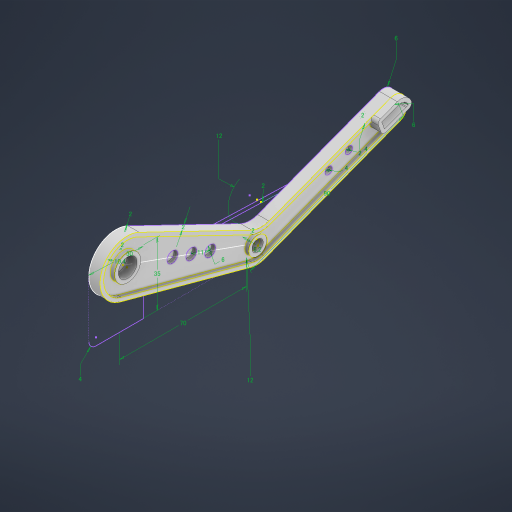
# Autodesk Inventor part: myPartbasic
Saved by Autodesk Inventor 2024.3 (Build 283343000, 343)
## iProperties
Created: 2024-11-22
Part Number: myPartbasic
Material: 一般
Document SubType Name: Modeling
Designer: ktamu
Density: 1 g/cm^3
Appearance: 既定
Author: ktamu
Autodesk Inventor part; units mm, degrees
ref_plane "YZ Plane" through (0, 0, 0) normal (1, 0, 0) x (0, 1, 0)
ref_plane "XZ Plane" through (0, 0, 0) normal (0, 1, 0) x (-1, 0, 0)
ref_plane "XY Plane" through (0, 0, 0) normal (0, 0, 1) x (1, 0, 0)
sketch "スケッチ1" plane through (0, 0, 0) normal (1, 0, 0) x (0, 1, 0)
  circle A0 centre (0, 0) radius 5.2
  circle A1 centre (0, 0) radius 7.2
  circle A2 centre (0, 0) radius 15
  line L0 (0, 15) -> (0, -15)
  line L1 (0, -15) -> (-35, -15)
  line L2 (-35, -15) -> (-35, 11)
  line L3 (-31, 15) -> (0, 15) construction
  line L4 (-35, -2) -> (-35, -69.78961) construction
  line L5 (-16.456445, -68.521985) -> (13.505431, -6.527122)
  line L6 (-34.785535, -71.500897) -> (-3.071406, -155.728054) construction
  line L7 (-16.882388, -77.972233) -> (8.360316, -145.012424)
  line L8 (4.859448, -152.741843) -> (2.520189, -153.622646)
  arc A3 (-16.456445, -68.521985) -> (-16.882388, -77.972233) centre (-5.6521, -73.743683) ccw
  line L9 (-11.514893, -58.297296) -> (-12.535445, -89.51695)
  line L10 (-9.368656, -53.856465) -> (-10.694227, -94.406903)
  arc A4 (-31, 15) -> (-35, 11) centre (-31, 11) ccw
  line L11 (-33.982617, -68.236115) -> (-14.480338, 3.914053)
  line L12 (-33.610765, -75.643066) -> (-5.200295, -150.145356)
  arc A5 (-33.982617, -68.236115) -> (-33.610765, -75.643066) centre (-22.398347, -71.367357) ccw
  circle A6 centre (-25.713339, -72) radius 3.1
  circle A7 centre (-25.713339, -72) radius 5.1
  circle A8 centre (0, 0) radius 13
  arc A9 (4.859448, -152.741843) -> (8.360316, -145.012424) centre (2.745173, -147.126699) ccw
  arc A10 (-5.200295, -150.145356) -> (2.520189, -153.622646) centre (0.405914, -148.007502) ccw
  line L13 (11.704707, -5.656839) -> (-18.257169, -67.651702)
  arc A11 (-18.257169, -67.651702) -> (-18.754102, -78.676992) centre (-5.6521, -73.743683) ccw
  line L14 (-18.754102, -78.676992) -> (6.488602, -145.717182)
  arc A12 (4.154689, -150.870128) -> (6.488602, -145.717182) centre (2.745173, -147.126699) ccw
  line L15 (4.154689, -150.870128) -> (1.815431, -151.750931)
  arc A13 (-3.331559, -149.432738) -> (1.815431, -151.750931) centre (0.405914, -148.007502) ccw
  line L16 (-3.331559, -149.432738) -> (-31.742028, -74.930447)
  arc A14 (-32.051905, -68.757988) -> (-31.742028, -74.930447) centre (-22.398347, -71.367357) ccw
  line L17 (-32.051905, -68.757988) -> (-12.549626, 3.392179)
  line L18 (4.154689, -133.843017) -> (-1.799139, -136.084817)
  line L19 (-2.966095, -138.66129) -> (1.944291, -151.702412)
  arc A15 (-1.799139, -136.084817) -> (-2.966095, -138.66129) centre (-1.09438, -137.956532) ccw
  line L20 (4.859448, -135.714731) -> (-1.09438, -137.956532)
  line L21 (-1.09438, -137.956532) -> (3.816005, -150.997653)
  line L22 (1.944291, -151.702412) -> (2.649049, -153.574126)
  line L23 (3.816005, -150.997653) -> (4.520764, -152.869368)
  arc A16 (1.944291, -151.702412) -> (4.520764, -152.869368) centre (4.117287, -150.332466) ccw
  arc A17 (3.31554, -149.668506) -> (4.859448, -150.522261) centre (4.408491, -149.5149) ccw
  point P0 (-35, -72)
  point P1 (-12.549626, 3.392179)
  point P2 (3.485655, -150.1203)
  point P3 (2.987733, -136.41949)
  dimension "d0" = 10.4
  dimension "d1" = 2
  dimension "d2" = 30
  dimension "d3" = 35
  dimension "d4" = 70
  dimension "d6" = 90
  dimension "d8" = 12
  dimension "d9" = 2
  dimension "d10" = 4
  dimension "d11" = 12
  dimension "d12" = 6.2
  dimension "d13" = 2
  dimension "d14" = 2
  dimension "d15" = 6
  dimension "d16" = 6
  dimension "d17" = 2
  dimension "d26" = 2
  dimension "d27" = 2
  constraints: 48 end point, 29 point on circle, 18 centre point, 14 point on line, 14 tangent, 7 perpendicular, 5 coincident, 4 parallel, 2 vertical, 1 midpoint, 9 other
  measures "d0" diameter of A0
  measures "d1" radial gap between concentric circles of A1 A0
  measures "d2" diameter of A2
  measures "d3" distance of L0.end L1.end
  measures "d4" distance of L4.start point (-35, -72)
  measures "d6" distance of L6.start L6.end
  measures "d8" radius of A3
  measures "d9" distance between parallel lines of L10 L9
  measures "d10" radius of A4
  measures "d11" radius of A5
  measures "d12" diameter of A6
  measures "d13" radial gap between concentric circles of A7 A6
  measures "d14" radial gap between concentric circles of A2 A8
  measures "d15" radius of A9
  measures "d16" radius of A10
  measures "d17" distance between parallel lines of L5 L13
  measures "d26" radius of A15
  measures "d27" distance between parallel lines of L18 L20
extrude "押し出し1" add sketch "スケッチ1" along normal blind 6.2 contours A8 L17 A2 L0 | L0 A2 L13 A8 | A2 L17 L1 L11 | A2 L5 A3 L7 L18 L14 A11 L13 | L17 A14 L16 A13 L15 L22 L8 A10 L12 A5 L11 L1 | L18 L7 L20 L14 | L20 L7 A9 L8 L23 L15 A12 L14 | A16 L8 L22 | L15 L23 A16 picked at (-13.999587, -0.567157) picked at (10.206953, -9.598345)
extrude "押し出し2" add sketch "スケッチ1" along normal blind 6.5 contours A0 L0 A1 | A0 L0 A1
extrude "押し出し3" add sketch "スケッチ1" along normal blind 4 contours L0 A8 A1 | A1 L0 A8 | A8 L13 A2 L0 | L0 A2 L17 A8 | L1 L17 A2 | A2 L13 A11 L14 L18 A15 L19 L15 A13 L16 A14 L17 L1 | L14 L20 L21 A17 L15 L19 A15 L18 | L14 A12 A17 L21 L20 | A12 L15 L21 A17 | L21 A17 picked at (7.393067, -11.426958) picked at (-1.085027, -14.214185)
extrude "押し出し4" add sketch "スケッチ1" along normal blind 6 contours A7
sketch "スケッチ2" plane through (6.2, 0, 0) normal (1, 0, 0) x (0, 0, -1)
  arc A0 (68.236115, -33.982617) -> (75.643066, -33.610765) centre (71.367357, -22.398347) ccw
  line L0 (75.643066, -33.610765) -> (150.145356, -5.200295)
  arc A1 (150.145356, -5.200295) -> (153.622646, 2.520189) centre (148.007502, 0.405914) ccw
  line L1 (153.622646, 2.520189) -> (152.741843, 4.859448)
  arc A2 (152.741843, 4.859448) -> (145.012424, 8.360316) centre (147.126699, 2.745173) ccw
  line L2 (145.012424, 8.360316) -> (77.972233, -16.882388)
  arc A3 (68.521985, -16.456445) -> (77.972233, -16.882388) centre (73.743683, -5.6521) ccw
  line L3 (68.521985, -16.456445) -> (6.527122, 13.505431)
  arc A4 (6.527122, 13.505431) -> (-3.914053, -14.480338) centre (0, 0) ccw
  line L4 (-3.914053, -14.480338) -> (68.236115, -33.982617)
  line L5 (68.757988, -32.051905) -> (-3.392179, -12.549626)
  arc A5 (5.656839, 11.704707) -> (-3.392179, -12.549626) centre (0, 0) ccw
  line L6 (5.656839, 11.704707) -> (67.651702, -18.257169)
  arc A6 (67.651702, -18.257169) -> (78.676992, -18.754102) centre (73.743683, -5.6521) ccw
  line L7 (78.676992, -18.754102) -> (145.717182, 6.488602)
  arc A7 (150.870128, 4.154689) -> (145.717182, 6.488602) centre (147.126699, 2.745173) ccw
  line L8 (150.870128, 4.154689) -> (151.750931, 1.815431)
  arc A8 (149.432738, -3.331559) -> (151.750931, 1.815431) centre (148.007502, 0.405914) ccw
  line L9 (149.432738, -3.331559) -> (74.930447, -31.742028)
  arc A9 (68.757988, -32.051905) -> (74.930447, -31.742028) centre (71.367357, -22.398347) ccw
  line L10 (68.757988, -32.051905) -> (-3.392179, -12.549626)
  arc A10 (68.757988, -32.051905) -> (74.930447, -31.742028) centre (71.367357, -22.398347) ccw
  line L11 (149.432738, -3.331559) -> (74.930447, -31.742028)
  arc A11 (149.432738, -3.331559) -> (151.750931, 1.815431) centre (148.007502, 0.405914) ccw
  line L12 (150.870128, 4.154689) -> (151.750931, 1.815431)
  arc A12 (150.870128, 4.154689) -> (145.717182, 6.488602) centre (147.126699, 2.745173) ccw
  line L13 (78.676992, -18.754102) -> (145.717182, 6.488602)
  arc A13 (67.651702, -18.257169) -> (78.676992, -18.754102) centre (73.743683, -5.6521) ccw
  line L14 (5.656839, 11.704707) -> (67.651702, -18.257169)
  arc A14 (5.656839, 11.704707) -> (-3.392179, -12.549626) centre (0, 0) ccw
  circle A15 centre (0, 0) radius 7.2
  circle A16 centre (72, -25.713339) radius 5.1
extrude "押し出し5" add sketch "スケッチ1" along normal blind 10 contours L18 L7 L20 L14 | L14 L20 L21 A17 L15 L19 A15 L18 | L20 L7 A9 L8 L23 L15 A12 L14 | L15 L23 A16
fillet "フィレット1" radius 2 1 edges at (8.1, 4.1547, -133.843)
sketch "スケッチ3" plane through (4, -2.966095, -138.66129) normal (0, -0.9358573, -0.3523792) x (1, 0, 0)
  circle A0 centre (4, -7.182404) radius 1.047988
  line L0 (0, -13.934947) -> (0, 0)
  line L1 (2.2, -13.934947) -> (0, -13.934947)
  line L2 (2.2, -13.934947) -> (6, -13.934947)
  line L3 (6, 0) -> (6, -13.934947)
  line L4 (0, 0) -> (6, 0)
  point P0 (-4, 128.721991)
  dimension "d31" = 2
  constraints: 1 centre point
  measures "d31" distance from line of L3 A0.centre
extrude "押し出し6" cut sketch "スケッチ3" against normal blind 1.25 contours A0
sketch "スケッチ4" plane through (4, 0, 0) normal (1, 0, 0) x (0, 0, -1)
  line L0 (151.702412, 1.944291) -> (138.66129, -2.966095)
  arc A0 (136.084817, -1.799139) -> (138.66129, -2.966095) centre (137.956532, -1.09438) ccw
  line L1 (136.084817, -1.799139) -> (134.547775, 2.282975)
  line L2 (78.676992, -18.754102) -> (134.547775, 2.282975)
  arc A1 (67.651702, -18.257169) -> (78.676992, -18.754102) centre (73.743683, -5.6521) ccw
  line L3 (5.656839, 11.704707) -> (67.651702, -18.257169)
  arc A2 (5.656839, 11.704707) -> (-3.392179, -12.549626) centre (0, 0) ccw
  line L4 (68.757988, -32.051905) -> (-3.392179, -12.549626)
  arc A3 (68.757988, -32.051905) -> (74.930447, -31.742028) centre (71.367357, -22.398347) ccw
  line L5 (149.432738, -3.331559) -> (74.930447, -31.742028)
  arc A4 (149.432738, -3.331559) -> (151.750931, 1.815431) centre (148.007502, 0.405914) ccw
  line L6 (151.702412, 1.944291) -> (151.750931, 1.815431)
  circle A5 centre (0, 0) radius 7.2
  circle A6 centre (72, -25.713339) radius 5.1
  circle A7 centre (72, -25.713339) radius 3.1
  line L7 (0, 0) -> (72, -25.713339)
  circle A8 centre (47.784268, -17.065182) radius 3
  circle A9 centre (124.237326, -7.2) radius 2
  circle A10 centre (113.080305, -11.373416) radius 2
  circle A11 centre (37.425064, -13.365602) radius 3
  circle A12 centre (27.06586, -9.666023) radius 3
  dimension "d34" = 6
  dimension "d35" = 4
  dimension "d36" = 4
  dimension "d41" = 11
  constraints: 5 centre point, 2 end point, 1 point on line, 5 other
  measures "d34" diameter of A8
  measures "d35" diameter of A9
  measures "d36" diameter of A10
  measures "d41" distance of A8.centre A11.centre
extrude "押し出し7" cut sketch "スケッチ4" against normal blind 2 contours A8 L7 | L7 A8 | A9 | A10
extrude "押し出し8" cut sketch "スケッチ4" against normal blind 2 contours A12 L7 | L7 A12 | A11 L7 | L7 A11
extrude "押し出し9" add sketch "スケッチ1" along normal blind 1 contours A0 L0 | L0 A0
extrude "押し出し10" add sketch "スケッチ1" along normal blind 1 contours A6
